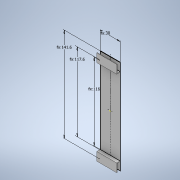
# Autodesk Inventor part: coil_spacer
Saved by Autodesk Inventor 2021 (Build 250183000, 183)
## iProperties
Created: 2021-02-09
Part Number: coil_spacer
Material: Generic
Document SubType Name: Modeling
Designer: pduy110
Density: 1 g/cm^3
Appearance: Default
Author: pduy110
Autodesk Inventor part; units mm, degrees
ref_plane "YZ Plane" through (0, 0, 0) normal (1, 0, 0) x (0, 1, 0)
ref_plane "XZ Plane" through (0, 0, 0) normal (0, 1, 0) x (-1, 0, 0)
ref_plane "XY Plane" through (0, 0, 0) normal (0, 0, 1) x (1, 0, 0)
sketch "Sketch1" plane through (0, 0, 0) normal (0, 0, 1) x (1, 0, 0)
  line L0 (-15, 70.8) -> (15, 70.8)
  line L1 (15, 70.8) -> (15, -70.8)
  line L2 (15, -70.8) -> (-15, -70.8)
  line L3 (-15, -70.8) -> (-15, 70.8)
  line L4 (0, 70.8) -> (0, -70.8) construction
  line L5 (-15, 58.8) -> (15, 58.8)
  line L6 (15, 58.8) -> (15, -58.8)
  line L7 (15, -58.8) -> (-15, -58.8)
  line L8 (-15, -58.8) -> (-15, 58.8)
  line L9 (0, 58.8) -> (0, -58.8) construction
  line L10 (-15, 58) -> (15, 58)
  line L11 (15, 58) -> (15, -58)
  line L12 (15, -58) -> (-15, -58)
  line L13 (-15, -58) -> (-15, 58)
  line L14 (0, 58) -> (0, -58) construction
  point P0 (0, 0)
  point P1 (0, 0)
  point P2 (15, -58)
  point P3 (-15, -58)
  point P4 (-15, -58.8)
  point P5 (15, -58.8)
  point P6 (-15, 58)
  point P7 (15, 58)
  point P8 (15, 58.8)
  point P9 (-15, 58.8)
  dimension "d0" = 141.6
  dimension "d1" = 30
  dimension "d4" = 117.6
  dimension "d5" = 116
  constraints: 30 end point, 9 midpoint, 6 parallel, 3 horizontal, 3 perpendicular, 2 coincident, 2 collinear
  measures "d0" distance between parallel lines of L2 L0
  measures "d1" distance between parallel lines of L1 L3
  measures "d4" distance between parallel lines of L7 L5
  measures "d5" distance between parallel lines of L12 L10
extrude "Extrusion1" add sketch "Sketch1" against normal blind 0.6
extrude "Extrusion2" add sketch "Sketch1" along normal blind 5.2 contours L5 L1 L10 L3 | L12 L1 L7 L3
ref_plane "upper Plane" through (0, 0, 5.2) normal (0, 0, 1) x (1, 0, 0)
sketch "Sketch2" plane through (0, 0, 5.2) normal (0, 0, 1) x (1, 0, 0)
  line L0 (-15, 70.8) -> (15, 70.8) projected
  line L1 (-15, 70.8) -> (-15, 58.8) projected
  line L2 (-15, 58) -> (-15, -58) projected
  line L3 (-15, -58) -> (-15, -58.8) projected
  line L4 (-15, -58.8) -> (-15, -70.8) projected
  line L5 (-15, -70.8) -> (15, -70.8) projected
  line L6 (15, -70.8) -> (15, -58.8) projected
  line L7 (15, -58.8) -> (15, -58) projected
  line L8 (15, -58) -> (15, 58) projected
  line L9 (15, 58.8) -> (15, 70.8) projected
  line L10 (15, 58) -> (15, 58.8) projected
  line L11 (-15, 58.8) -> (-15, 58) projected
  line L12 (15, 58.8) -> (-15, 58.8) projected
  line L13 (-15, -58.8) -> (15, -58.8) projected
  point P0 (0, 0)
extrude "Extrusion4" add sketch "Sketch2" against normal blind 0.6 contours L0 L9 L12 L1 | L13 L6 L5 L4
equation "\"d0\" = coil_spacer_width + 2 * grab_distance"
equation "\"d1\" = coil_spacer_length"
equation "\"d4\" = coil_spacer_width"
equation "\"d5\" = coil_spacer_width - 2 * wire_diameter_tolerance"
equation "\"d2\" = coil_spacer_thickness"
equation "\"d6\" = wire_diameter"
equation "\"d11\" = coil_spacer_thickness"
equation "\"coil_spacer_length\" = 30"
equation "\"coil_spacer_width\" = 117.6"
equation "\"coil_spacer_thickness\" = 0.6"
equation "\"grab_distance\" = 12"
equation "\"wire_diameter_tolerance\" = 0.8"
equation "\"wire_diameter\" = 5.2"
body "Solid1"
